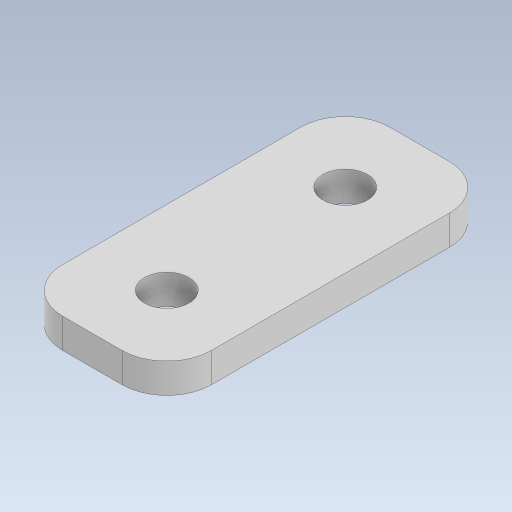
# Autodesk Inventor part: Konektor Casis 2
Saved by Autodesk Inventor 2023.5 (Build 275446000, 446)
## iProperties
Created: 2025-09-16
Part Number: Konektor Casis 2
Material: Generic
Document SubType Name: Modeling
Designer: Guntur
Density: 1 g/cm^3
Appearance: Default
Author: Guntur
## iProperties of the stored document Konektor Casis 2_3DPrint.ipt
Created: 2025-09-21
Part Number: Konektor Casis 2_3DPrint
Material: Generic
Document SubType Name: Modeling
Designer: Guntur
Density: 1 g/cm^3
Appearance: Default
Author: Guntur
Autodesk Inventor part; units mm, degrees
ref_plane "YZ Plane" through (0, 0, 0) normal (1, 0, 0) x (0, 1, 0)
ref_plane "XZ Plane" through (0, 0, 0) normal (0, 1, 0) x (-1, 0, 0)
ref_plane "XY Plane" through (0, 0, 0) normal (0, 0, 1) x (1, 0, 0)
sketch "Sketch1" plane through (0, 0, 0) normal (0, 1, 0) x (-1, 0, 0)
  line L0 (1.5875, 0) -> (-2.17, 0) construction
  line L1 (0, 2.1822) -> (0, -1.8687) construction
  circle A0 centre (0, 6) radius 1.5
  line L2 (0, 11) -> (2, 11)
  line L3 (5, 8) -> (5, 0)
  arc A1 (5, 8) -> (2, 11) centre (2, 8) ccw
  line L4 (0, 11) -> (-2, 11)
  line L5 (-5, 8) -> (-5, 0)
  arc A2 (-2, 11) -> (-5, 8) centre (-2, 8) ccw
  circle A3 centre (0, -6) radius 1.5
  line L6 (0, -11) -> (2, -11)
  line L7 (5, -8) -> (5, 0)
  arc A4 (2, -11) -> (5, -8) centre (2, -8) ccw
  line L8 (-5, -8) -> (-5, 0)
  arc A5 (-5, -8) -> (-2, -11) centre (-2, -8) ccw
  line L9 (0, -11) -> (-2, -11)
  point P0 (0, 0)
  point P1 (5, 11)
  point P2 (-5, 11)
  point P3 (5, -11)
  point P4 (-5, -11)
  dimension "d0" = 3
  dimension "d1" = 6
  dimension "d2" = 5
  dimension "d3" = 5
  dimension "d4" = 3
  constraints: 20 end point, 15 symmetric about line, 8 point on circle, 8 point on line, 6 centre point, 3 horizontal, 3 vertical, 2 tangent, 5 other
  measures "d0" diameter of A0
  measures "d1" distance from line of L0 A0.centre
  measures "d2" distance of L2.start point (5, 11)
  measures "d3" distance from line of L2 A0.centre
  measures "d4" radius of A1
extrude "Extrusion1" add sketch "Sketch1" along normal blind 2
body "Solid1"
